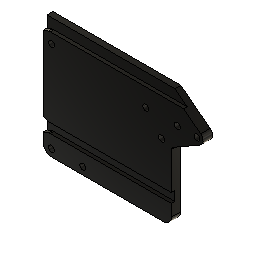
ThrowerStatorSidePlate v6 (Autodesk Fusion 360 design; units mm, degrees)
Autodesk Fusion 360 part; units mm, degrees
sketch "Sketch1" plane through (0, 0, 0) normal (0, 1, 0) x (1, 0, 0)
  circle A0 centre (0, 0) radius 48 construction
  circle A1 centre (0, 0) radius 14 construction
  circle A2 centre (0, 0) radius 9.5 construction
  circle A3 centre (0, 0) radius 8 construction
  line L0 (0, 0) -> (8, 0) construction
  line L1 (0, 0) -> (0, -9.5) construction
  line L2 (0, 0) -> (-8, 0) construction
  line L3 (0, 0) -> (0, 9.5) construction
  circle A4 centre (8, 0) radius 1.5
  circle A5 centre (-8, 0) radius 1.5
  circle A6 centre (0, 9.5) radius 1.5
  circle A7 centre (0, 0) radius 12 construction
  line L4 (8, 0) -> (18, 0) construction
  line L5 (21.1, 0) -> (19.55, 2.6847) construction
  line L6 (19.55, 2.6847) -> (16.45, 2.6847) construction
  line L7 (16.45, 2.6847) -> (14.9, 0) construction
  line L8 (14.9, 0) -> (16.45, -2.6847) construction
  line L9 (16.45, -2.6847) -> (19.55, -2.6847) construction
  line L10 (19.55, -2.6847) -> (21.1, 0) construction
  circle A8 centre (18, 0) radius 3.1 construction
  circle A9 centre (18, 0) radius 1.5
  line L11 (0, 52) -> (-68, 52) construction
  line L12 (-9.7468, 47) -> (-68, 47) construction
  line L13 (-68, 52) -> (-68, 47) construction
  line L14 (-68, 47) -> (-68, 35.633) construction
  line L15 (-68, 35.633) -> (-32.1604, 35.633) construction
  line L16 (-68, 35.633) -> (-68, 30.833) construction
  line L17 (-68, 30.833) -> (-36.7876, 30.833) construction
  line L18 (-68, 30.833) -> (-68, -9.167) construction
  line L19 (-60, -9.167) -> (-47.1165, -9.167)
  line L20 (-68, -9.167) -> (-68, -13.967) construction
  line L21 (-68, -13.967) -> (-45.923, -13.967) construction
  line L22 (-60, -13.967) -> (-60, 35.633)
  line L23 (5.9333, 10.4305) -> (19.5328, 2.6945)
  line L24 (-60, -13.967) -> (21.1, -13.967)
  line L25 (21.1, -13.967) -> (21.1, 0)
  arc A10 (21.1, 0) -> (19.5328, 2.6945) centre (18, 0) ccw
  line L26 (-57, 35.633) -> (5, 35.633)
  line L27 (5, 35.633) -> (5, 11.8322)
  arc A11 (5.9333, 10.4305) -> (5.7778, 10.5175) centre (0, 0) ccw
  arc A12 (5, 11.8322) -> (5.7778, 10.5175) centre (6.5, 11.8322) ccw
  arc A13 (5.7778, 10.5175) -> (7.9656, 11.513) centre (6.5, 11.8322) ccw construction
  arc A14 (5.4445, 12.898) -> (5, 11.8322) centre (6.5, 11.8322) ccw construction
  arc A15 (7.9656, 11.513) -> (5.4445, 12.898) centre (6.5, 11.8322) ccw construction
  line L28 (5, 11.8322) -> (5, 10.9087) construction
  arc A16 (5.7778, 10.5175) -> (5, 10.9087) centre (0, 0) ccw construction
  line L29 (-57, 30.833) -> (5, 30.833)
  line L30 (-47.1165, -9.167) -> (21.1, -9.167)
  line L31 (-60, 35.633) -> (-60, 45.633)
  line L32 (-60, 45.633) -> (5, 45.633)
  line L33 (5, 45.633) -> (5, 35.633)
  circle A17 centre (-56, 42) radius 1.5
  circle A18 centre (-40, 42) radius 1.5
  line L34 (-40, 42) -> (0, 0) construction
  circle A19 centre (-55.8448, -4.167) radius 1.5
  line L35 (0, 0) -> (-55.8448, -4.167) construction
  line L36 (-68, -9.167) -> (-60, -9.167) construction
  line L37 (-57, -9.167) -> (-60, -8.167)
  line L38 (-57, -9.167) -> (-57, 30.833) construction
  line L39 (-57, 30.833) -> (-57, 35.633) construction
  line L40 (-57, 30.833) -> (-60, 29.833)
  line L41 (-57, 35.633) -> (-60, 36.633)
  line L42 (-60, 35.633) -> (-57, 35.633) construction
  line L43 (-60, 30.833) -> (-57, 30.833) construction
  line L44 (5, 11.8322) -> (5, -13.967) construction
  line L45 (5, -13.967) -> (19.8959, -2.4527)
  line L46 (18, 0) -> (19.8959, -2.4527) construction
  line L47 (18, 0) -> (21.1, 0) construction
  arc A20 (19.8959, -2.4527) -> (21.1, 0) centre (18, 0) ccw
  point P0 (18, 0)
  point P1 (-33.1034, 34.7586)
  point P2 (-47.8669, -3.5717)
  dimension "d1" = 96
  dimension "d2" = 28
  dimension "d3" = 19
  dimension "d4" = 16
  dimension "d5" = 3
  dimension "d6" = 3
  dimension "d7" = 3
  dimension "d8" = 24
  dimension "d9" = 18
  dimension "d10" = 3.1
  dimension "d11" = 60
  dimension "d12" = 3
  dimension "d13" = 52
  dimension "d14" = 68
  dimension "d15" = 68
  dimension "d18" = 5
  dimension "d22" = 16.367
  dimension "d23" = 4.8
  dimension "d24" = 40
  dimension "d25" = 4.8
  dimension "d26" = 8
  dimension "d27" = 3.1
  dimension "d28" = 5
  dimension "d33" = 12
  dimension "d34" = 3
  dimension "d35" = 10
  dimension "d36" = 3
  dimension "d37" = 12
  dimension "d38" = 5
  dimension "d39" = 3
  dimension "d40" = 5
  dimension "d41" = 10
  dimension "d42" = 3
  dimension "d43" = 5
  dimension "d44" = 8
  dimension "d54" = 1
  dimension "d55" = 3
  dimension "d56" = 1
  dimension "d57" = 1
  dimension "d60" = 3.1
  constraint coincident A0.centre A1.centre
  constraint concentric A1 A3
  constraint coincident A3 L0.end
  constraint horizontal L0
  constraint coincident A2 L1.end
  constraint perpendicular L0 L1
  constraint coincident A3 L2.end
  constraint perpendicular L1 L2
  constraint coincident A2 L3.end
  constraint perpendicular L2 L3
  constraint coincident L0.end A4.centre
  constraint coincident L2.end A5.centre
  constraint coincident L3.end A6.centre
  constraint concentric A2 A7
  constraint parallel L0 L4
  constraint coincident P0 L4.end
  constraint coincident L8.end A8
  constraint horizontal L11
  constraint coincident A0 L12.start
  constraint parallel L11 L12
  constraint perpendicular L12 L13
  constraint perpendicular L12 L14
  constraint coincident A0 L15.end
  constraint perpendicular L14 L15
  constraint perpendicular L15 L16
  constraint coincident A0 L17.end
  constraint perpendicular L16 L17
  constraint perpendicular L17 L18
  constraint coincident A0 L19.end
  constraint perpendicular L18 L19
  constraint perpendicular L19 L20
  constraint coincident A0 L21.end
  constraint perpendicular L20 L21
  constraint coincident L21 L22.start
  constraint coincident L15 L22.end
  constraint perpendicular L15 L22
  constraint coincident A7 L23.start
  constraint coincident A8 L23.end
  constraint tangent A8 L23
  constraint tangent A7 L23
  constraint perpendicular L22 L24
  constraint tangent A8 L25
  constraint perpendicular L22 L26
  constraint coincident A7 L28.end
  constraint vertical L27
  constraint tangent L27 A13
  constraint tangent A11 A13
  constraint coincident A7 A11.end
  constraint concentric A12 A13
  constraint coincident A1 A13.end
  constraint coincident A1 A14.start
  constraint concentric A13 A14
  constraint concentric A13 A15
  constraint vertical L28
  constraint concentric A11 A16
  constraint coincident L27 L29.end
  constraint perpendicular L27 L29
  constraint coincident L25 L30.end
  constraint perpendicular L25 L30
  constraint perpendicular L15 L31
  constraint perpendicular L27 L32
  constraint perpendicular L26 L33
  constraint coincident A18.centre L34.start
  constraint coincident A0 P1
  constraint coincident L34 P1
  constraint coincident A19.centre L35.end
  constraint coincident L35 P2
  constraint coincident A0 P2
  constraint coincident L22 L19.start
  constraint perpendicular L18 L36
  constraint coincident L22 L43.start
  constraint coincident L17.end L29
  constraint coincident L19 L37.start
  constraint coincident L22 L37.end
  constraint coincident L17 L29.start
  constraint coincident L15 L26.start
  constraint coincident L22 L40.end
  constraint coincident L31 L41.end
  constraint vertical L38
  constraint vertical L39
  constraint coincident L24 L44.end
  constraint tangent A12 L44
  constraint perpendicular L24 L44
  constraint coincident A8 L45.end
  constraint tangent A8 L45
  constraint perpendicular L25 L47
  measures "d1" diameter of A0
  measures "d2" diameter of A1
  measures "d3" diameter of A2
  measures "d4" diameter of A3
  measures "d5" diameter of A4
  measures "d6" diameter of A5
  measures "d7" diameter of A6
  measures "d8" diameter of A7
  measures "d9" distance of A0.centre P0
  measures "d10" distance of L5.start P0
  measures "d11" angle of L4 L8
  measures "d12" diameter of A9
  measures "d13" distance of A0.centre L11
  measures "d14" horizontal distance of A0.centre L11.end
  measures "d15" distance of L11.start L11.end
  measures "d18" distance of L11 L12
  measures "d22" distance of L11 L15
  measures "d23" distance of L14.end L16.end
  measures "d24" distance of L16.end L18.end
  measures "d25" distance of L18.end L20.end
  measures "d26" distance of L18 L22
  measures "d27" radius of A10
  measures "d28" horizontal distance of A0.centre L26.end
  measures "d33" radius of A11
  measures "d34" diameter of A13
  measures "d35" distance of L15 L32
  measures "d36" diameter of A17
  measures "d37" distance of L14 A17.centre
  measures "d38" distance of L12 A17.centre
  measures "d39" diameter of A18
  measures "d40" distance of L12 A18.centre
  measures "d41" distance of A18.centre P1
  measures "d42" diameter of A19
  measures "d43" distance of L19 A19.centre
  measures "d44" distance of A19.centre P2
  measures "d54" distance of L19.start L37.end
  measures "d55" distance of L31 L26.start
  measures "d56" distance of L22.end L41.end
  measures "d57" distance of L43.start L40.end
  measures "d60" radius of A20
extrude "Extrude1" add sketch "Sketch1" along normal blind 4.8 contours L19 L22 L37 | L19 L22 L24 L30 L45 | L19 L22 L23 A10 L27 A11 A12 L29 L30 L37 L40 L45 A20 | L22 L26 L27 L29 L31 L40 L41 | L26 L31 L32 L33 L41
fillet "Fillet1" radius 4 2 edges at (5, 2.4, -45.633) (-60, 2.4, -45.633)
extrude "Extrude2" cut sketch "Sketch1" along normal blind 1.8 contours L19 L22 L37 | L19 L22 L24 L30 L45 | L22 L26 L27 L29 L31 L40 L41
fillet "Fillet2" radius 3 3 edges at (-57, 0.9, -35.633) (-57, 0.9, -30.833) (-57, 0.9, 9.167)
